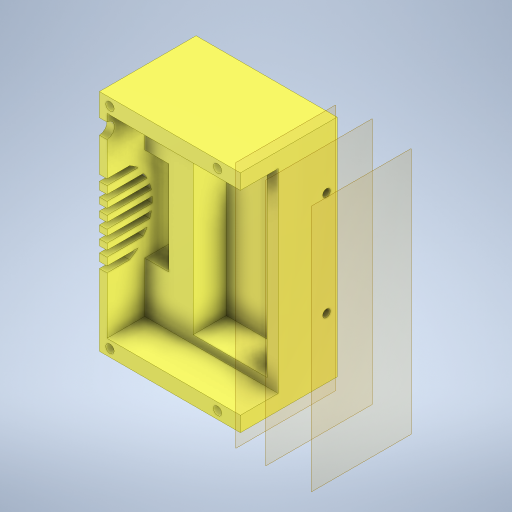
# Autodesk Inventor part: caseLowerPortionBack
Saved by Autodesk Inventor 2023 (Build 270158030, 158C)
## iProperties
Created: 2021-08-20
Part Number: caseLowerPortionBack
Material: PC/ABS Plastic
Document SubType Name: Modeling
Designer: robst
Density: 0.357273 g/cm^3
Appearance: Smooth - Yellow
Author: robst
Autodesk Inventor part; units mm, degrees
ref_plane "XZ Plane" through (0, 0, 0) normal (0, 1, 0) x (-1, 0, 0)
ref_plane "XY Plane" through (0, 0, 0) normal (0, 0, 1) x (1, 0, 0)
sketch "Sketch1" plane through (0, 0, 0) normal (0, 0, 1) x (1, 0, 0)
  line L0 (-111.35, -74.5) -> (111.35, -74.5)
  line L1 (111.35, -74.5) -> (111.35, 74.5)
  line L2 (111.35, 74.5) -> (-111.35, 74.5)
  line L3 (-111.35, 74.5) -> (-111.35, -74.5)
  line L4 (-111.35, -74.5) -> (111.35, 74.5) construction
  line L5 (111.35, -74.5) -> (-111.35, 74.5) construction
  point P0 (0, 0)
  dimension "d0" = 222.7
  dimension "d1" = 149
  constraints: 12 end point, 2 midpoint, 2 parallel, 1 horizontal, 1 perpendicular
  measures "d0" distance of L0.start L0.end
  measures "d1" distance of L1.end L0.end
extrude "MainInnerBodyExtrusion" add sketch "Sketch1" against normal blind 50
sketch "Sketch3" plane through (0, 0, 0) normal (0, 0, 1) x (1, 0, 0)
  line L0 (36.65, -27) -> (95.65, -27)
  line L1 (95.65, -27) -> (95.65, 27)
  line L2 (95.65, 27) -> (36.65, 27)
  line L3 (36.65, 27) -> (36.65, -27)
  line L4 (36.65, -27) -> (95.65, 27) construction
  line L5 (95.65, -27) -> (36.65, 27) construction
  line L6 (111.35, -74.5) -> (111.35, 74.5) projected
  line L7 (0, 0) -> (111.35, 0) construction
  line L8 (-111.35, -74.5) -> (-111.35, 74.5) construction
  line L9 (-111.35, 74.5) -> (-111.35, -74.5) projected
  point P0 (66.15, 0)
  point P1 (66.15, 0)
  dimension "d5" = 15.7
  dimension "d6" = 54
  dimension "d7" = 59
  constraints: 14 end point, 4 midpoint, 2 parallel, 1 horizontal, 1 perpendicular, 1 point on line
  measures "d5" distance between parallel lines of L1 L6
  measures "d6" distance of L0.end L1.end
  measures "d7" distance of L1.end L2.end
extrude "HoleForCamerabase" cut sketch "Sketch3" against normal blind 47
sketch "Sketch4" plane through (0, 0, 0) normal (0, 0, 1) x (1, 0, 0)
  line L0 (0, 0) -> (-111.35, 0) construction
  line L1 (-111.35, -74.5) -> (-111.35, 74.5) construction
  line L2 (-108.35, -31) -> (-92.35, -31)
  line L3 (-92.35, -31) -> (-92.35, 31)
  line L4 (-92.35, 31) -> (-108.35, 31)
  line L5 (-108.35, 31) -> (-108.35, -31)
  line L6 (-108.35, -31) -> (-92.35, 31) construction
  line L7 (-92.35, -31) -> (-108.35, 31) construction
  point P0 (-100.35, 0)
  dimension "d13" = 16
  dimension "d14" = 62
  dimension "d15" = 3
  constraints: 14 end point, 3 midpoint, 2 parallel, 1 perpendicular, 1 point on line
  measures "d13" distance of L2.start L2.end
  measures "d14" distance of L3.end L2.end
  measures "d15" distance between parallel lines of L1 L5
extrude "HoleForFan" cut sketch "Sketch4" against normal blind 47
sketch "Sketch6" plane through (0, 0, 0) normal (0, 0, 1) x (1, 0, 0)
  line L0 (-111.35, -74.5) -> (-111.35, 74.5) construction
  line L1 (-111.35, 0) -> (111.35, 0) construction
  line L2 (111.35, 74.5) -> (111.35, -74.5) construction
  line L3 (-11.35, -64.5) -> (20.65, -64.5)
  line L4 (20.65, -64.5) -> (20.65, 64.5)
  line L5 (20.65, 64.5) -> (-11.35, 64.5)
  line L6 (-11.35, 64.5) -> (-11.35, -64.5)
  line L7 (-11.35, -64.5) -> (20.65, 64.5) construction
  line L8 (20.65, -64.5) -> (-11.35, 64.5) construction
  line L9 (36.65, -27) -> (36.65, 27) projected
  point P0 (0, 0)
  point P1 (4.65, 0)
  dimension "d20" = 32
  dimension "d21" = 129
  dimension "d88" = 16
  constraints: 14 end point, 4 midpoint, 3 parallel, 1 perpendicular, 1 point on line
  measures "d20" distance of L3.start L3.end
  measures "d21" distance of L4.end L3.end
  measures "d88" distance between parallel lines of L4 L9
extrude "HoleForPi" cut sketch "Sketch6" against normal blind 47
sketch "Sketch7" plane through (0, 0, 0) normal (0, 0, 1) x (1, 0, 0)
  line L0 (0, 0) -> (-111.35, 0) construction
  line L1 (-111.35, 74.5) -> (-111.35, -74.5) construction
  line L2 (-76.35, -59) -> (-27.35, -59)
  line L3 (-27.35, -59) -> (-27.35, 59)
  line L4 (-27.35, 59) -> (-76.35, 59)
  line L5 (-76.35, 59) -> (-76.35, -59)
  line L6 (-76.35, -59) -> (-27.35, 59) construction
  line L7 (-27.35, -59) -> (-76.35, 59) construction
  line L8 (-11.35, -64.5) -> (-11.35, 64.5) projected
  line L9 (-92.35, 31) -> (-92.35, -31) construction
  point P0 (-51.85, 0)
  dimension "d25" = 16
  dimension "d26" = 49
  dimension "d27" = 118
  constraints: 14 end point, 3 midpoint, 2 parallel, 1 perpendicular, 1 point on line
  measures "d25" distance between parallel lines of L3 L8
  measures "d26" distance of L2.start L2.end
  measures "d27" distance of L4.end L2.start
extrude "HoleForPoeAdapter" cut sketch "Sketch7" against normal blind 47
sketch "Sketch10" plane through (0, 0, 0) normal (0, 0, 1) x (1, 0, 0)
  line L0 (39.35, 36.5) -> (108.35, 36.5)
  line L1 (108.35, 36.5) -> (108.35, 64.5)
  line L2 (108.35, 64.5) -> (39.35, 64.5)
  line L3 (39.35, 64.5) -> (39.35, 36.5)
  line L4 (39.35, 36.5) -> (108.35, 64.5) construction
  line L5 (108.35, 36.5) -> (39.35, 64.5) construction
  line L6 (111.35, 74.5) -> (-111.35, 74.5) projected
  line L7 (111.35, -74.5) -> (111.35, 74.5) projected
  point P0 (0, 0)
  point P1 (73.85, 50.5)
  point P2 (94.85, 8.5)
  point P3 (108.35, 50.5)
  dimension "d36" = 69
  dimension "d37" = 28
  dimension "d85" = 3
  constraints: 12 end point, 3 midpoint, 2 parallel, 1 horizontal, 1 perpendicular, 1 other
  measures "d36" distance of L1.end L2.end
  measures "d37" distance of L0.end L1.end
extrude "HoleForThermister" cut sketch "Sketch10" against normal blind 47
sketch "Sketch11" plane through (0, 0, 0) normal (0, 0, 1) x (1, 0, 0)
  line L0 (58.35, -64.5) -> (108.35, -64.5)
  line L1 (108.35, -64.5) -> (108.35, -47.5)
  line L2 (108.35, -47.5) -> (58.35, -47.5)
  line L3 (58.35, -47.5) -> (58.35, -64.5)
  line L4 (58.35, -64.5) -> (108.35, -47.5) construction
  line L5 (108.35, -64.5) -> (58.35, -47.5) construction
  line L6 (111.35, -74.5) -> (111.35, 74.5) projected
  line L7 (-111.35, -74.5) -> (111.35, -74.5) projected
  line L8 (95.65, -27) -> (36.65, -27) projected
  line L9 (20.65, 64.5) -> (20.65, -64.5) projected
  point P0 (0, 0)
  point P1 (83.35, -56)
  point P2 (94.85, -8.5)
  point P3 (83.35, -47.5)
  point P4 (58.35, -56)
  point P5 (111.35, 74.5)
  dimension "d42" = 50
  dimension "d43" = 17
  dimension "d86" = 3
  dimension "d87" = 10
  constraints: 12 end point, 4 midpoint, 2 parallel, 1 horizontal, 1 perpendicular, 1 other
  measures "d42" distance of L0.start L0.end
  measures "d43" distance of L0.end L1.end
  measures "d87" distance between parallel lines of L7 L0
extrude "HoleForSensor" cut sketch "Sketch11" against normal blind 31.5
sketch "Sketch15" plane through (-111.35, -74.5, 0) normal (-1, 0, 0) x (0, 0, 1)
  line L0 (0, 149) -> (0, 0) projected
  line L1 (0, 149) -> (-50, 149) projected
  line L2 (-50, 0) -> (-50, 149) projected
  line L3 (0, 0) -> (-50, 0) projected
  line L4 (0, 0) -> (0, 149) projected
  line L5 (0, 101.5) -> (0, 47.5) projected
  line L6 (0, 74.5) -> (-30, 74.5) construction
  line L7 (0, 76.5) -> (-29.9333, 76.5)
  line L8 (0, 84.5) -> (-28.2843, 84.5)
  line L9 (0, 80.5) -> (-29.3939, 80.5)
  line L10 (0, 76.5) -> (0, 74.5)
  line L11 (0, 88.5) -> (-26.533, 88.5)
  line L12 (0, 92.5) -> (-24, 92.5)
  line L13 (-20.5913, 97.5) -> (0, 97.5)
  line L14 (-14.9666, 101.5) -> (0, 101.5)
  line L15 (0, 84.5) -> (0, 80.5)
  line L16 (0, 101.5) -> (0, 97.5)
  line L17 (0, 92.5) -> (0, 88.5)
  line L18 (0, 72.5) -> (-29.9333, 72.5)
  line L19 (0, 64.5) -> (-28.2843, 64.5)
  line L20 (0, 68.5) -> (-29.3939, 68.5)
  line L21 (0, 72.5) -> (0, 74.5)
  line L22 (0, 60.5) -> (-26.533, 60.5)
  line L23 (0, 56.5) -> (-24, 56.5)
  line L24 (-20.5913, 51.5) -> (0, 51.5)
  line L25 (-14.9666, 47.5) -> (0, 47.5)
  line L26 (0, 64.5) -> (0, 68.5)
  line L27 (0, 56.5) -> (0, 60.5)
  line L28 (0, 47.5) -> (0, 51.5)
  line L29 (0, 72.5) -> (0, 76.5)
  line L30 (0, 80.5) -> (0, 84.5)
  line L31 (0, 88.5) -> (0, 92.5)
  line L32 (0, 97.5) -> (0, 149)
  arc A0 (-28.2843, 84.5) -> (-29.3939, 80.5) centre (0, 74.5) ccw
  arc A1 (-14.9666, 101.5) -> (-20.5913, 97.5) centre (0, 74.5) ccw
  arc A2 (-24, 92.5) -> (-26.533, 88.5) centre (0, 74.5) ccw
  arc A3 (-29.9333, 76.5) -> (-29.9333, 72.5) centre (0, 74.5) ccw
  arc A4 (-29.3939, 68.5) -> (-28.2843, 64.5) centre (0, 74.5) ccw
  arc A5 (-26.533, 60.5) -> (-24, 56.5) centre (0, 74.5) ccw
  arc A6 (-20.5913, 51.5) -> (-14.9666, 47.5) centre (0, 74.5) ccw
  point P0 (0, 82)
  point P1 (0, 67.0167)
  point P2 (0, 4.25)
  point P3 (-10.2956, 97.5)
  point P4 (0, 47.5)
  point P5 (0, 51.5)
  point P6 (0, 56.5)
  point P7 (0, 60.5)
  point P8 (0, 64.5)
  point P9 (0, 68.5)
  point P10 (0, 72.5)
  point P11 (0, 80.5)
  point P12 (0, 84.5)
  point P13 (0, 88.5)
  point P14 (0, 92.5)
  point P15 (0, 97.5)
  point P16 (0, 101.5)
  dimension "d69" = 2
  dimension "d71" = 4
  dimension "d72" = 4
  dimension "d73" = 4
  dimension "d75" = 4
  dimension "d142" = 30
  constraints: 54 end point, 15 point on circle, 15 symmetric about line, 7 centre point, 3 parallel, 3 perpendicular, 2 horizontal, 1 coincident, 1 midpoint, 1 other
  measures "d69" distance between parallel lines of L7 L6
  measures "d71" distance between parallel lines of L8 L9
  measures "d72" distance between parallel lines of L11 L8
  measures "d73" distance between parallel lines of L12 L11
  measures "d75" distance between parallel lines of L13 L14
  measures "d142" radius of A2
extrude "SlotsForRearFan" cut sketch "Sketch15" against normal up to surface (3 mm away) contours L0 L13 A1 L14 | L0 L11 A2 L12 | L25 A6 L24 L0 | L0 L9 A0 L8 | L23 A5 L22 L0 | L0 L18 A3 L7 | L19 A4 L20 L0
sketch "Sketch16" plane through (0, 0, -47) normal (0, 0, 1) x (1, 0, 0)
  line L0 (95.65, 27) -> (95.65, -27) projected
  line L1 (80.15, 10.765) -> (80.15, -11.235) construction
  line L2 (78.65, 10.765) -> (78.65, -11.235)
  line L3 (75.65, -11.235) -> (75.65, 10.765)
  line L4 (72.65, 8.7746) -> (72.65, -9.2446)
  line L5 (69.65, 3.5785) -> (69.65, -4.0485)
  line L6 (81.65, 10.765) -> (81.65, -11.235)
  line L7 (84.65, -11.235) -> (84.65, 10.765)
  line L8 (87.65, 8.7746) -> (87.65, -9.2446)
  line L9 (90.65, 3.5785) -> (90.65, -4.0485)
  line L10 (73.7991, 10.765) -> (75.65, 10.765)
  line L11 (75.65, -11.235) -> (73.7991, -11.235)
  line L12 (73.7991, -11.235) -> (72.65, -9.2446)
  line L13 (69.65, -4.0485) -> (67.4483, -0.235)
  line L14 (67.4483, -0.235) -> (69.65, 3.5785)
  line L15 (72.65, 8.7746) -> (73.7991, 10.765)
  line L16 (78.65, 10.765) -> (81.65, 10.765)
  line L17 (84.65, 10.765) -> (86.5009, 10.765)
  line L18 (86.5009, -11.235) -> (84.65, -11.235)
  line L19 (81.65, -11.235) -> (78.65, -11.235)
  line L20 (92.8517, -0.235) -> (90.65, -4.0485)
  line L21 (87.65, -9.2446) -> (86.5009, -11.235)
  line L22 (86.5009, 10.765) -> (87.65, 8.7746)
  line L23 (90.65, 3.5785) -> (92.8517, -0.235)
  point P0 (0, 0)
  point P1 (80.15, -0.235)
  point P2 (69.65, -0.235)
  dimension "d78" = 15.5
  dimension "d89" = 1.5
  dimension "d90" = 3
  dimension "d91" = 3
  dimension "d92" = 3
  constraints: 46 end point, 8 symmetric about line, 6 perpendicular, 3 horizontal, 3 midpoint, 2 vertical, 7 other
  measures "d78" distance from line of point (80.15, -0.235) L0
  measures "d89" distance between parallel lines of L2 L1
  measures "d90" distance between parallel lines of L3 L2
  measures "d91" distance between parallel lines of L4 L3
  measures "d92" distance from line of point (69.65, -0.235) L4
extrude "VentForCamera" cut sketch "Sketch16" against normal through all
sketch "Sketch18" plane through (111.35, -74.5, 0) normal (1, 0, 0) x (0, 0, -1)
  line L0 (0, 74.5) -> (29.6767, 74.5) construction
  arc A0 (24, 66.5) -> (24, 82.5) centre (24, 74.5) ccw
  line L1 (0, 0) -> (0, 149) projected
  line L2 (24, 82.5) -> (0, 82.5)
  line L3 (24, 66.5) -> (0, 66.5)
  line L4 (0, 82.5) -> (0, 66.5)
  point P0 (0, 74.5)
  dimension "d97" = 16
  dimension "d137" = 24
  constraints: 8 end point, 3 point on line, 2 perpendicular, 2 point on circle, 2 tangent, 1 centre point, 1 collinear, 1 horizontal, 1 midpoint
  measures "d97" diameter of A0
  measures "d137" distance of point (0, 74.5) A0.centre
extrude "HoleForLens" cut sketch "Sketch18" against normal up to surface (15.7 mm away)
sketch "Sketch23" plane through (0, 0, 0) normal (0, 0, 1) x (1, 0, 0)
  line L0 (-106.35, -69.5) -> (106.35, -69.5) construction
  line L1 (106.35, -69.5) -> (106.35, 69.5) construction
  line L2 (106.35, 69.5) -> (-106.35, 69.5) construction
  line L3 (-106.35, 69.5) -> (-106.35, -69.5) construction
  line L4 (-106.35, -69.5) -> (106.35, 69.5) construction
  line L5 (106.35, -69.5) -> (-106.35, 69.5) construction
  line L6 (111.35, -74.5) -> (111.35, -8) projected
  line L7 (111.35, 74.5) -> (-111.35, 74.5) projected
  line L8 (-111.35, -27) -> (-111.35, -74.5) projected
  line L9 (-111.35, 74.5) -> (-111.35, 27) projected
  line L10 (111.35, 8) -> (111.35, 74.5) projected
  point P0 (0, 0)
  point P1 (35.15, -69.5)
  point P2 (-35.15, -69.5)
  point P3 (-35.15, 69.5)
  point P4 (35.15, 69.5)
  dimension "d106" = 5
  dimension "d108" = 5
  dimension "d222" = 76.2
  dimension "d223" = 76.2
  dimension "d224" = 76.2
  dimension "d225" = 76.2
  constraints: 12 end point, 4 coincident, 4 point on line, 2 midpoint, 2 parallel, 1 horizontal, 1 perpendicular
  measures "d106" distance between parallel lines of L1 L6
  measures "d108" distance between parallel lines of L2 L7
  measures "d222" distance from line of point (35.15, -69.5) L6
  measures "d223" distance from line of point (-35.15, -69.5) L8
  measures "d224" distance from line of point (-35.15, 69.5) L9
  measures "d225" distance from line of point (35.15, 69.5) L10
hole "Hole for 6-32 Insert" at (-106.35, 69.5, 0) at (106.35, 69.5, 0) at (106.35, -69.5, 0) at (-106.35, -69.5, 0) at (-35.15, -69.5, 0) at (35.15, -69.5, 0) at (-35.15, 69.5, 0) at (35.15, 69.5, 0) direction (0, 0, -1) diameter 4.7 depth 7.2 tip angle 118 counterbore diameter 5.54 counterbore depth 5.55
hole "Screw hole for 6-32 screw" at (-106.35, -69.5, 0) at (106.35, -69.5, 0) at (106.35, 69.5, 0) at (-106.35, 69.5, 0) direction (0, 0, -1) diameter 3.797 depth 15 tip angle 118 clearance for "Hex Machine Screw" size "#6" standard "Ansi Unified Screw Threads"
sketch "Sketch24" plane through (-111.35, -74.5, 0) normal (0, -1, 0) x (1, 0, 0)
  line L0 (0, -50) -> (222.7, -50) construction
  line L1 (222.7, 0) -> (207, 0) construction
  line L2 (0, 0) -> (0, -50) projected
  line L3 (111.3501, -25) -> (0, -25) construction
  line L4 (111.3501, -25) -> (222.7, -24.84) construction
  line L5 (222.7, 0) -> (222.7, -50) construction
  point P0 (111.35, 0)
  dimension "d226" = 25
  dimension "d227" = 111.3501
  constraints: 4 end point, 1 equal length, 1 midpoint, 1 point on line, 2 other
  measures "d226" distance between parallel lines of L3 L0
  measures "d227" distance from line of L3.start L2
hole "Side hole for 1-4 20 insert" at (0.0001, -74.5, -25) direction (0, 1, 0) diameter 7.666 depth 9.53 tip angle 118 counterbore diameter 8.406 counterbore depth 7.41 clearance for "Hex Machine Screw" size "1/4" standard "Ansi Unified Screw Threads"
mirror "Mirror for side insert" about plane through (0, 0, 0) normal (0, 1, 0) of "Side hole for 1-4 20 insert"
sketch "Sketch25" plane through (0, 0, 0) normal (0, 0, 1) x (1, 0, 0)
  line L0 (111.35, 74.5) -> (-111.35, 74.5) projected
  line L1 (-111.35, 74.5) -> (-111.35, 27) projected
  line L2 (-111.35, -74.5) -> (111.35, -74.5) projected
  line L3 (81.65, -11.235) -> (78.65, -11.235) projected
  line L4 (78.65, -11.235) -> (78.65, 10.765) projected
  line L5 (78.65, 10.765) -> (81.65, 10.765) projected
  line L6 (81.65, 10.765) -> (81.65, -11.235) projected
  line L7 (73.7991, 10.765) -> (75.65, 10.765) projected
  line L8 (75.65, 10.765) -> (75.65, -11.235) projected
  line L9 (75.65, -11.235) -> (73.7991, -11.235) projected
  line L10 (73.7991, -11.235) -> (72.65, -9.2446) projected
  line L11 (72.65, -9.2446) -> (72.65, 8.7746) projected
  line L12 (72.65, 8.7746) -> (73.7991, 10.765) projected
  line L13 (87.65, 8.7746) -> (87.65, -9.2446) projected
  line L14 (87.65, -9.2446) -> (86.5009, -11.235) projected
  line L15 (86.5009, -11.235) -> (84.65, -11.235) projected
  line L16 (84.65, -11.235) -> (84.65, 10.765) projected
  line L17 (84.65, 10.765) -> (86.5009, 10.765) projected
  line L18 (86.5009, 10.765) -> (87.65, 8.7746) projected
  line L19 (69.65, 3.5785) -> (69.65, -4.0485) projected
  line L20 (69.65, -4.0485) -> (67.4483, -0.235) projected
  line L21 (67.4483, -0.235) -> (69.65, 3.5785) projected
  line L22 (92.8517, -0.235) -> (90.65, -4.0485) projected
  line L23 (90.65, -4.0485) -> (90.65, 3.5785) projected
  line L24 (90.65, 3.5785) -> (92.8517, -0.235) projected
  line L25 (95.65, 27) -> (95.65, -27) projected
  line L26 (36.65, 27) -> (95.65, 27) projected
  line L27 (36.65, -27) -> (36.65, 27) projected
  line L28 (95.65, -27) -> (36.65, -27) projected
  line L29 (111.35, -74.5) -> (111.35, -8) projected
  line L30 (111.35, 8) -> (111.35, 74.5) projected
  line L31 (-108.35, -64.5) -> (108.35, -64.5)
  line L32 (108.35, -64.5) -> (108.35, 64.5)
  line L33 (108.35, 64.5) -> (-108.35, 64.5)
  line L34 (-108.35, 64.5) -> (-108.35, -64.5)
  line L35 (-108.35, -64.5) -> (108.35, 64.5) construction
  line L36 (108.35, -64.5) -> (-108.35, 64.5) construction
  line L37 (-27.35, 59) -> (-27.35, -59) projected
  point P0 (0, 0)
  dimension "d138" = 10
  dimension "d139" = 3
  constraints: 12 end point, 2 midpoint, 2 parallel, 2 perpendicular
  measures "d138" distance between parallel lines of L2 L31
  measures "d139" distance between parallel lines of L1 L34
extrude "Extrusion18" cut sketch "Sketch25" against normal blind 25 contours L34 L33 L32 L31
sketch "Sketch26" plane through (-111.35, -74.5, -50) normal (-1, 0, 0) x (0, 0, 1)
  arc A0 (50, 124) -> (50, 134) centre (50, 129) ccw
  circle A1 centre (50, 129) radius 5
  point P0 (50, 74.5)
  point P1 (50, 124)
  constraints: 2 centre point, 2 point on circle, 1 coincident, 1 concentric, 4 other
extrude "Extrusion19" cut sketch "Sketch26" against normal up to surface (3 mm away)
sketch "Sketch30" plane through (111.35, -74.5, -50) normal (1, 0, 0) x (0, 0, -1)
  circle A0 centre (-29, 74.5) radius 27.5
  line L0 (0, 149) -> (0, 0) projected
  circle A1 centre (-29, 74.5) radius 23
  line L1 (-50, 0) -> (-50, 66.5) projected
  point P0 (-50, 74.5)
  dimension "poeLength" = 118
  dimension "d162" = 55
  dimension "d163" = 29
  dimension "d164" = 46
  dimension "d165" = 21
  constraints: 2 centre point, 1 coincident
  measures "d162" diameter of A0
  measures "d163" distance from line of L0 A0.centre
  measures "d164" diameter of A1
  measures "d165" distance from line of L1 A0.centre
extrude "Extrusion20" cut sketch "Sketch30" against normal blind 1.5
sketch "Sketch35" plane through (111.35, -74.5, -50) normal (1, 0, 0) x (0, 0, -1)
  circle A0 centre (-13, 5) radius 2.4257
  circle A1 centre (-13, 144) radius 2.4257
  line L0 (-50, 0) -> (0, 0) projected
  line L1 (-50, 149) -> (0, 149) projected
  line L2 (-3, 139) -> (-3, 10) projected
  point P0 (-50, 74.5)
  dimension "d215" = 4.8514
  dimension "d216" = 5
  dimension "d217" = 5
  dimension "d218" = 10
  dimension "d219" = 10
  constraints: 2 centre point, 1 equal radius
  measures "d215" diameter of A1
  measures "d216" distance from line of A0.centre L0
  measures "d217" distance from line of A1.centre L1
  measures "d218" distance from line of A0.centre L2
  measures "d219" distance from line of A1.centre L2
extrude "Extrusion21" cut sketch "Sketch35" against normal blind 9.525
sketch "Sketch37" plane through (-111.35, -74.5, -50) normal (-1, 0, 0) x (0, 0, 1)
  arc A0 (50, 134) -> (50, 124) centre (50, 129) ccw projected
  line L0 (50, 149) -> (50, 134) projected
  line L1 (50, 149) -> (0, 149) projected
  line L2 (0, 0) -> (0, 149) projected
  line L3 (50, 0) -> (0, 0) projected
  line L4 (50, 47.5) -> (50, 0) projected
  line L5 (50, 47.5) -> (35.0334, 47.5) projected
  arc A1 (29.4087, 51.5) -> (35.0334, 47.5) centre (50, 74.5) ccw projected
  line L6 (29.4087, 51.5) -> (50, 51.5) projected
  line L7 (50, 56.5) -> (50, 51.5) projected
  line L8 (50, 56.5) -> (26, 56.5) projected
  arc A2 (23.467, 60.5) -> (26, 56.5) centre (50, 74.5) ccw projected
  line L9 (23.467, 60.5) -> (50, 60.5) projected
  line L10 (50, 64.5) -> (50, 60.5) projected
  line L11 (50, 64.5) -> (21.7157, 64.5) projected
  arc A3 (20.6061, 68.5) -> (21.7157, 64.5) centre (50, 74.5) ccw projected
  line L12 (20.6061, 68.5) -> (50, 68.5) projected
  line L13 (50, 72.5) -> (50, 68.5) projected
  line L14 (50, 72.5) -> (20.0667, 72.5) projected
  arc A4 (20.0667, 76.5) -> (20.0667, 72.5) centre (50, 74.5) ccw projected
  line L15 (20.0667, 76.5) -> (50, 76.5) projected
  line L16 (50, 80.5) -> (50, 76.5) projected
  line L17 (50, 80.5) -> (20.6061, 80.5) projected
  arc A5 (21.7157, 84.5) -> (20.6061, 80.5) centre (50, 74.5) ccw projected
  line L18 (21.7157, 84.5) -> (50, 84.5) projected
  line L19 (50, 88.5) -> (50, 84.5) projected
  line L20 (50, 88.5) -> (23.467, 88.5) projected
  arc A6 (26, 92.5) -> (23.467, 88.5) centre (50, 74.5) ccw projected
  line L21 (26, 92.5) -> (50, 92.5) projected
  line L22 (50, 97.5) -> (50, 92.5) projected
  line L23 (50, 97.5) -> (29.4087, 97.5) projected
  arc A7 (35.0334, 101.5) -> (29.4087, 97.5) centre (50, 74.5) ccw projected
  line L24 (35.0334, 101.5) -> (50, 101.5) projected
  line L25 (50, 124) -> (50, 101.5) projected
  line L26 (0, 149) -> (50, 149)
  line L27 (50, 149) -> (50, 0)
  line L28 (50, 0) -> (0, 0)
  line L29 (0, 0) -> (0, 149)
  constraints: 8 end point, 2 parallel, 1 horizontal, 1 perpendicular
extrude "Extrusion22" add sketch "Sketch37" along normal blind 2 contours A0 L25 L24 A7 L23 L22 L21 A6 L20 L19 L18 A5 L17 L16 L15 A4 L14 L13 L12 A3 L11 L10 L9 A2 L8 L7 L6 A1 L5 L4 L3 L2 L1 L0
sketch "Sketch38" plane through (111.35, -74.5, -50) normal (1, 0, 0) x (0, 0, -1)
  circle A0 centre (-13, 144) radius 2.4257 projected
  circle A1 centre (-13, 5) radius 2.4257 projected
  arc A2 (-50, 56.7447) -> (-50, 92.2553) centre (-29, 74.5) ccw projected
  line L0 (-50, 0) -> (-50, 56.7447) projected
  line L1 (-50, 0) -> (0, 0) projected
  line L2 (0, 149) -> (0, 0) projected
  line L3 (-50, 149) -> (0, 149) projected
  line L4 (-50, 92.2553) -> (-50, 149) projected
  arc A3 (-50, 65.1192) -> (-50, 83.8808) centre (-29, 74.5) ccw projected
  line L5 (-26, 66.5) -> (-50, 66.5) projected
  arc A4 (-26, 66.5) -> (-26, 82.5) centre (-26, 74.5) ccw projected
  line L6 (-50, 82.5) -> (-26, 82.5) projected
  point P0 (-50, 74.5)
extrude "Extrusion23" add sketch "Sketch38" along normal blind 2
sketch "Sketch39" plane through (0, 0, -50) normal (0, 0, -1) x (-1, 0, 0)
  line L0 (-78.65, -11.235) -> (-81.65, -11.235) projected
  line L1 (-81.65, -11.235) -> (-81.65, 10.765) projected
  line L2 (-81.65, 10.765) -> (-78.65, 10.765) projected
  line L3 (-78.65, 10.765) -> (-78.65, -11.235) projected
  line L4 (-75.65, 10.765) -> (-73.7991, 10.765) projected
  line L5 (-73.7991, 10.765) -> (-72.65, 8.7746) projected
  line L6 (-72.65, 8.7746) -> (-72.65, -9.2446) projected
  line L7 (-72.65, -9.2446) -> (-73.7991, -11.235) projected
  line L8 (-73.7991, -11.235) -> (-75.65, -11.235) projected
  line L9 (-75.65, -11.235) -> (-75.65, 10.765) projected
  line L10 (-87.65, -9.2446) -> (-87.65, 8.7746) projected
  line L11 (-87.65, 8.7746) -> (-86.5009, 10.765) projected
  line L12 (-86.5009, 10.765) -> (-84.65, 10.765) projected
  line L13 (-84.65, 10.765) -> (-84.65, -11.235) projected
  line L14 (-84.65, -11.235) -> (-86.5009, -11.235) projected
  line L15 (-86.5009, -11.235) -> (-87.65, -9.2446) projected
  line L16 (-69.65, -4.0485) -> (-69.65, 3.5785) projected
  line L17 (-69.65, 3.5785) -> (-67.4483, -0.235) projected
  line L18 (-67.4483, -0.235) -> (-69.65, -4.0485) projected
  line L19 (-90.65, -4.0485) -> (-92.8517, -0.235) projected
  line L20 (-92.8517, -0.235) -> (-90.65, 3.5785) projected
  line L21 (-90.65, 3.5785) -> (-90.65, -4.0485) projected
  line L22 (113.35, -74.5) -> (-113.35, -74.5) projected
  line L23 (113.35, 74.5) -> (113.35, -74.5) projected
  line L24 (-113.35, 74.5) -> (113.35, 74.5) projected
  line L25 (-113.35, -74.5) -> (-113.35, 74.5) projected
  line L26 (113.35, -74.5) -> (-113.35, -74.5) projected
  line L27 (-113.35, 74.5) -> (113.35, 74.5)
  line L28 (113.35, 74.5) -> (113.35, -74.5)
  line L29 (113.35, -74.5) -> (-113.35, -74.5)
  line L30 (-113.35, -74.5) -> (-113.35, 74.5)
  point P0 (0, 0)
  constraints: 8 end point, 2 parallel, 1 horizontal, 1 perpendicular
extrude "ExtrusionForBottom" add sketch "Sketch39" along normal blind 14
sketch "Sketch40" plane through (113.35, -74.5, -50) normal (1, 0, 0) x (0, 0, -1)
  line L0 (-50, 0) -> (14, 0) construction
  line L1 (7, 0) -> (7, 149) construction
  line L2 (-50, 149) -> (14, 149) construction
  line L3 (14, 149) -> (14, 0) construction
  point P0 (-50, 74.5)
  point P1 (7, 40)
  point P2 (7, 109)
  dimension "d234" = 7
  dimension "d235" = 40
  dimension "d236" = 40
  constraints: 4 point on line, 2 end point, 1 vertical
  measures "d234" distance between parallel lines of L1 L3
  measures "d235" distance of point (7, 40) L1.start
  measures "d236" distance from line of point (7, 109) L2
hole "10-32 holesToBoltFixture" at (113.35, -34.5, -57) at (113.35, 34.5, -57) direction (-1, 0, 0) diameter 5.105 end through all counterbore diameter 13.335 counterbore depth 6.35 clearance for "Hex Machine Screw" size "#10" standard "Ansi Unified Screw Threads"
sketch "Sketch41" plane through (109.85, -74.5, -50) normal (1, 0, 0) x (0, 0, -1)
  arc A0 (-50, 56.7447) -> (-50, 92.2553) centre (-29, 74.5) ccw projected
  arc A1 (-50, 65.1192) -> (-50, 83.8808) centre (-29, 74.5) ccw projected
  line L0 (-50, 149) -> (14, 149) projected
  line L1 (-50, 149) -> (-50, 92.2553) projected
  arc A2 (-50, 56.7447) -> (-50, 92.2553) centre (-29, 74.5) ccw projected
  line L2 (-50, 56.7447) -> (-50, 0) projected
  line L3 (-50, 0) -> (14, 0) projected
  line L4 (14, 149) -> (14, 0) projected
  circle A3 centre (-13, 144) radius 2.4257 projected
  circle A4 centre (-13, 5) radius 2.4257 projected
  arc A5 (-50, 65.1192) -> (-50, 83.8808) centre (-29, 74.5) ccw
  arc A6 (-50, 56.7447) -> (-50, 92.2553) centre (-29, 74.5) ccw
  line L5 (-50, 56.5) -> (-50, 92.2553)
  circle A7 centre (7, 40) radius 6.6675 projected
  circle A8 centre (7, 109) radius 6.6675 projected
  point P0 (-50, 74.5)
  constraints: 4 point on circle, 3 point on line, 2 centre point, 2 coincident, 2 concentric, 2 end point, 1 vertical
extrude "Extrusion25" add sketch "Sketch41" along normal blind 2 contours L5 A1 A0
ref_plane "Work Plane1" through (30, 0, 0) normal (1, 0, 0) x (0, 1, 0)
ref_plane "Work Plane2" through (-20, 0, 0) normal (1, 0, 0) x (0, 1, 0)
mirror "Mirror4" about plane through (0, 0, 0) normal (1, 0, 0) of "10-32 holesToBoltFixture"
split "Split2" plane through (-20, 0, 0) removes the side toward (1, 0, 0)
equation "\"d0\" = newCaseLength"
equation "\"d1\" = caseWidth"
equation "\"d2\" = caseDepth"
equation "\"d5\" = lensLength"
equation "\"d6\" = cameraWidth"
equation "\"d7\" = cameraLength"
equation "\"d8\" = maxComponentDepth"
equation "\"d13\" = fanDepth"
equation "\"d14\" = fanWidth"
equation "\"d15\" = rearWallThickness"
equation "\"d16\" = maxComponentDepth"
equation "\"d20\" = piCaseDepth"
equation "\"d21\" = piCaseLength"
equation "\"d88\" = minDelta"
equation "\"d22\" = maxComponentDepth"
equation "\"d25\" = minDelta"
equation "\"d26\" = poeWidth"
equation "\"d27\" = poeLength"
equation "\"d28\" = maxComponentDepth"
equation "\"d36\" = thermisterLength"
equation "\"d37\" = thermisterWidth"
equation "\"d85\" = frontWallThickness"
equation "\"d38\" = maxComponentDepth"
equation "\"d42\" = sensorLength"
equation "\"d43\" = sensorWidth"
equation "\"d86\" = frontWallThickness"
equation "\"d87\" = outsideWallThickness"
equation "\"d46\" = cutoutDepth"
equation "\"outsideWallThickness\" = 10"
equation "\"caseWidth\" = piCaseLength + 2 * outsideWallThickness"
equation "\"cameraWidth\" = 54"
equation "\"oneHalfCaseDepth\" = piCaseWidth"
equation "\"caseLength\" = 189.7"
equation "\"cameraLength\" = 59"
equation "\"lensLength\" = 15.7"
equation "\"piCaseWidth\" = 63"
equation "\"piCaseDepth\" = 32"
equation "\"poeDepth\" = 38"
equation "\"piEthernetCableReliefLength\" = 35"
equation "\"poeEthernetCableReliefLength\" = 35"
equation "\"thermisterDepth\" = 18"
equation "\"sensorDepth\" = 11"
equation "\"cutoutDepth\" = 0.5 * piCaseWidth"
equation "\"thickenDistance\" = 1"
equation "\"bottomOfCaseWallThickness\" = 3"
equation "\"rearWallThickness\" = 3"
equation "\"maxComponentDepth\" = extraCutoutDepth + 0.5 * piCaseWidth"
equation "\"caseDepth\" = maxComponentDepth + bottomOfCaseWallThickness"
equation "\"minDelta\" = 16"
equation "\"fanCutoutDepth\" = 0.5 * fanLength + extraCutoutDepth + thickenDistance"
equation "\"newCaseLength\" = 222.7"
equation "\"frontWallThickness\" = 3"
equation "\"d95\" = lensDiameter"
equation "\"extraCutoutDepth\" = 15.5"
equation "\"bottomExtrusion\" = 14"
equation "\"fanDepth\" = 16"
equation "\"fanWidth\" = 62"
equation "\"piCaseLength\" = 129"
equation "\"poeWidth\" = 49"
equation "\"thermisterLength\" = 69"
equation "\"thermisterWidth\" = 28"
equation "\"sensorLength\" = 50"
equation "\"sensorWidth\" = 17"
equation "\"fanLength\" = 60"
equation "\"lensDiameter\" = 15"
body "Solid1"
